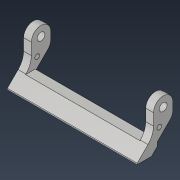
# Autodesk Inventor part: Chip Schaufel v2
Saved by Autodesk Inventor 2022.3 (Build 263350000, 350)
## iProperties
Part Number: Chip Schaufel v2
Material: Aluminium 6061
Document SubType Name: Modeling
Designer: rYan
Mass: 10.967 g
Surface Area: 30.2735 cm^2
Volume: 4.06184 cm^3
Density: 2.7 g/cm^3
Appearance: Aluminium - flach
Author: rYan
Autodesk Inventor part; units mm, degrees
ref_plane "YZ Plane" through (0, 0, 0) normal (1, 0, 0) x (0, 1, 0)
ref_plane "XZ Plane" through (0, 0, 0) normal (0, 1, 0) x (-1, 0, 0)
ref_plane "XY Plane" through (0, 0, 0) normal (0, 0, 1) x (1, 0, 0)
sketch "Skizze1" plane through (0, 0, 0) normal (1, 0, 0) x (0, 1, 0)
  line L0 (-4.8284, 6.1716) -> (-10.5, 0.5)
  line L1 (-10.5, 0) -> (-3, 0)
  line L2 (-10.5, 0.5) -> (-10.5, 0)
  line L3 (0, 5) -> (8, 13)
  circle A0 centre (3, 19) radius 0.5
  line L4 (-2, 13) -> (-2, 24)
  line L5 (-2, 24) -> (8, 24)
  line L6 (8, 24) -> (8, 13)
  line L7 (0, 3) -> (-3, 0)
  line L8 (8, 13) -> (-2, 13) construction
  arc A1 (-4.8284, 6.1716) -> (-2, 13) centre (-11.6569, 13) ccw
  line L9 (0, 5) -> (0, 3)
  line L10 (3, 19) -> (3, 0) construction
  point P0 (0, 0)
  dimension "d40" = 0.5
  dimension "d44" = 1
  dimension "d59" = 10
  dimension "d60" = 45
  dimension "d61" = 5
  dimension "d63" = 45
  dimension "d78" = 3
  dimension "d79" = 10.5
  dimension "d80" = 0
  dimension "d81" = 19
  dimension "d82" = 5
  dimension "d83" = 3
  constraints: 22 end point, 5 vertical, 2 centre point, 2 horizontal, 2 point on circle, 2 tangent, 1 parallel, 1 perpendicular, 1 point on line, 1 other
  measures "d40" distance of L0.end L1.start
  measures "d44" diameter of A0
  measures "d59" distance of L4.end L5.end
  measures "d60" angle of L7 L1
  measures "d61" distance from line of L3.start L1
  measures "d63" angle of L0 L1
  measures "d78" distance of point (0, 0) L1.end
  measures "d79" distance from line of point (0, 0) L2
  measures "d80" distance from line of point (0, 0) L9
  measures "d81" vertical distance of point (0, 0) L10.start
  measures "d82" distance from line of L5 L10.start
  measures "d83" horizontal distance of point (0, 0) L10.start
extrude "Extrusion1" add sketch "Skizze1" along normal mid plane 67
sketch "Skizze6" plane through (0, 0, 0) normal (0, 1, 0) x (-1, 0, 0)
  line L0 (33.5, 0.5) -> (-33.5, 0.5) projected
  line L1 (-33.5, 6.1716) -> (-33.5, 0.5) projected
  line L2 (33.5, 0.5) -> (33.5, 6.1716) projected
  line L3 (-29.5, 6) -> (29.5, 6)
  line L4 (29.5, 6) -> (29.5, 36)
  line L5 (29.5, 36) -> (-29.5, 36)
  line L6 (-29.5, 36) -> (-29.5, 6)
  line L7 (0, -7.2) -> (0, 43.2) projected
  line L8 (33.5, 0) -> (-33.5, 0) projected
  line L9 (-33.5, 0) -> (33.5, 0) projected
  point P0 (0, 0)
  point P1 (-33, 10)
  point P2 (33, 10)
  dimension "d45" = 4
  dimension "d46" = 30
  dimension "d50" = 6
  constraints: 8 end point, 2 parallel, 1 horizontal, 1 perpendicular, 3 other
  measures "d46" distance of L3.end L4.end
  measures "d50" distance between parallel lines of L8 L3
extrude "Extrusion4" cut sketch "Skizze6" along normal through all both and the other way through all
sketch "Skizze3" plane through (-33.5, 0, 0) normal (-1, 0, 0) x (0, 0, 1)
  line L0 (0, -3) -> (0, -10.5) projected
  line L1 (0.5, -10.5) -> (6.1716, -4.8284) projected
  line L2 (0, -10.5) -> (0, 0) construction
  line L3 (0, 11.9314) -> (0, -15.5882) projected
  line L4 (0, -10.5) -> (0.5, -10.5) projected
  line L5 (13, 8) -> (5, 0) projected
  line L6 (13, -2) -> (24, -2) projected
  line L7 (24, -2) -> (24, 8) projected
  line L8 (24, 8) -> (13, 8) projected
  circle A0 centre (19, 3) radius 0.5 projected
  line L9 (3, 0) -> (0, -3) projected
  arc A1 (13, -2) -> (6.1716, -4.8284) centre (13, -11.6569) ccw projected
  line L10 (5, 0) -> (3, 0) projected
  constraints: 1 coincident
hole "Bohrung1" at (-33.5, 3, 19) direction (1, 0, 0) diameter 4.05 end through all
sketch "Skizze4" plane through (-33.5, 0, 0) normal (-1, 0, 0) x (0, 0, 1)
  line L0 (0, 11.7) -> (0, -14.2) projected
  line L1 (-5.8, 0) -> (34.8, 0) projected
  point P0 (29, 0)
  point P1 (11, 1)
  dimension "d38" = 11
  dimension "d84" = 1
  measures "d38" distance from line of point (11, 1) L0
  measures "d84" distance from line of point (11, 1) L1
hole "Bohrung2" at (-33.5, 1, 11) direction (1, 0, 0) diameter 2.459 end through all thread size "M3x0.5" class "6H" standard "ISO Metric profile"
fillet "Rundung2" radius 5 6 edges at (31.5, -2, 24) (31.5, 8, 24) (-31.5, 8, 24) (-31.5, -2, 24) (31.5, 8, 13) (-31.5, 8, 13)
fillet "Rundung7" [suppressed]
fillet "Rundung8" radius 0.36 2 edges at (0, -10.5, 0.5) (0, -10.5, 0)
sketch "Skizze7" plane through (-29.5, 1, 6) normal (0, 0, 1) x (1, 0, 0)
  line L0 (0, 0) -> (59, 0) projected
  line L1 (0, 0) -> (0, -6) projected
  line L2 (59, -6) -> (0, -6) projected
  line L3 (59, -6) -> (59, 0) projected
  line L4 (-17.4, -1) -> (76.4, -1) projected
  point P0 (29.5, -1)
  point P1 (0, -1)
  point P2 (59, -1)
extrude "Extrusion5" cut sketch "Skizze7" against normal through all contours L0 L3 L4 L1
